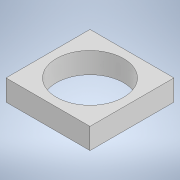
# Autodesk Inventor part: pipe2cube
Saved by Autodesk Inventor 2020 (Build 240168000, 168)
## iProperties
Created: 2023-02-14
Part Number: pipe2cube
Material: 一般
Document SubType Name: Modeling
Designer: satolab
Density: 1 g/cm^3
Appearance: 既定
Author: satolab
Autodesk Inventor part; units mm, degrees
ref_plane "YZ Plane" through (0, 0, 0) normal (1, 0, 0) x (0, 1, 0)
ref_plane "XZ Plane" through (0, 0, 0) normal (0, 1, 0) x (-1, 0, 0)
ref_plane "XY Plane" through (0, 0, 0) normal (0, 0, 1) x (1, 0, 0)
sketch "スケッチ1" plane through (0, 0, 0) normal (0, 1, 0) x (-1, 0, 0)
  circle A0 centre (0, 0) radius 16
  line L0 (20, 20) -> (-20, 20)
  line L1 (-20, 20) -> (-20, -20)
  line L2 (-20, -20) -> (20, -20)
  line L3 (20, -20) -> (20, 20)
  dimension "d0" = 32
  dimension "d1" = 20
  dimension "d2" = 20
  dimension "d3" = 20
  dimension "d4" = 20
  constraints: 8 end point, 2 parallel, 1 centre point, 1 coincident, 1 horizontal, 1 perpendicular
  measures "d0" diameter of A0
  measures "d1" distance from line of L2 A0.centre
  measures "d2" distance from line of A0.centre L0
  measures "d3" distance from line of point (0, 0) L3
  measures "d4" distance from line of point (0, 0) L1
extrude "押し出し1" add sketch "スケッチ1" along normal mid plane 10
